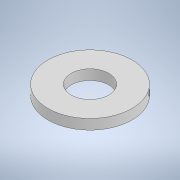
# Autodesk Inventor part: filwasher
Saved by Autodesk Inventor 2020 (Build 240168000, 168)
## iProperties
Created: 2019-07-05
Part Number: filwasher
Material: Generic
Document SubType Name: Modeling
Designer: ColinP
Density: 1 g/cm^3
Appearance: Default
Author: ColinP
Autodesk Inventor part; units mm, degrees
ref_plane "YZ Plane" through (0, 0, 0) normal (1, 0, 0) x (0, 1, 0)
ref_plane "XZ Plane" through (0, 0, 0) normal (0, 1, 0) x (-1, 0, 0)
ref_plane "XY Plane" through (0, 0, 0) normal (0, 0, 1) x (1, 0, 0)
sketch "Sketch1" plane through (0, 0, 0) normal (0, 1, 0) x (-1, 0, 0)
  circle A0 centre (0, 0) radius 1.4224
  circle A1 centre (0, 0) radius 3.175
  dimension "d0" = 2.8448
  dimension "d1" = 6.35
  constraints: 2 centre point, 2 coincident
  measures "d0" diameter of A0
  measures "d1" diameter of A1
extrude "Extrusion1" add sketch "Sketch1" along normal blind 0.762
sketch "Sketch2" plane through (0, 0, 0) normal (0, 0, 1) x (1, 0, 0)
  point P0 (0, 0)
sketch "Sketch3" plane through (0, 0, 0) normal (0, 1, 0) x (-1, 0, 0)
  point P0 (0, 0)
sketch "Sketch4" plane through (0, 0, 0) normal (1, 0, 0) x (0, 1, 0)
  line L0 (0.762, -3.175) -> (0.762, 3.175) projected
  line L1 (0.762, 0) -> (0, 0)
  line L2 (0, 0) -> (0.381, 0)
  line L3 (0, -3.175) -> (0.762, -3.175) projected
  line L4 (0.381, -3.175) -> (0.381, 0)
  line L5 (0.381, 3.1988) -> (0.381, 0)
  circle A0 centre (0.381, -2.0789) radius 0.1905
  dimension "d4" = 0.381
  constraints: 8 end point, 3 midpoint, 2 point on line, 1 centre point, 1 collinear, 1 horizontal, 1 perpendicular
  measures "d4" diameter of A0
extrude "Extrusion2" cut sketch "Sketch4" along normal through all both and the other way through all contours A0 L4 | L4 A0
body "Solid1"
